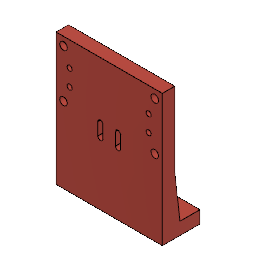
Y-endstop-holder-III-rev1 v6 (Autodesk Fusion 360 design; units mm, degrees)
Autodesk Fusion 360 part; units mm, degrees
note: some values were not read from the file. Set by a fixed rule: which sketch regions a step uses.
sketch "Sketch1" plane through (0, 0, 0) normal (0, 1, 0) x (1, 0, 0)
  line L0 (-21.15, 5) -> (21.15, 5)
  line L1 (21.15, 5) -> (21.15, -10)
  line L2 (21.15, -10) -> (-21.15, -10)
  line L3 (-21.15, -10) -> (-21.15, 5)
  line L4 (-15.5, 0) -> (15.5, 0) construction
  circle A0 centre (-15.5, 0) radius 1.5
  circle A1 centre (15.5, 0) radius 1.5
  circle A2 centre (0, 15.5) radius 14
  dimension "d1" = 42.3
  dimension "d2" = 15
  dimension "d3" = 31
  dimension "d4" = 5.65
  dimension "d5" = 3
  dimension "d6" = 3
  dimension "d9" = 28
  dimension "d13" = 15.5
  dimension "d14" = 5
  measures "d4" distance of origin
  measures "d5" diameter of A0
  measures "d6" diameter of A1
  measures "d9" diameter of A2
  measures "d14" distance of L0
extrude "Extrude1" add sketch "Sketch1" along normal blind 5 contours L0 L1 L2 L3 A2
sketch "Sketch2" plane through (0, 5, 0) normal (0, 1, 0) x (-1, 0, 0)
  line L0 (21.15, 5) -> (-21.15, 5)
  line L1 (-21.15, 5) -> (-21.15, 10)
  line L2 (-21.15, 10) -> (21.15, 10)
  line L3 (21.15, 10) -> (21.15, 5)
  circle A0 centre (-15.5, 0) radius 1.5
  circle A1 centre (15.5, 0) radius 1.5
  line L4 (-21.15, 10) -> (-21.15, -5)
  line L5 (-21.15, -5) -> (-9.2601, -5)
  arc A2 (9.2601, -5) -> (-9.2601, -5) centre (0, -15.5) ccw
  line L6 (9.2601, -5) -> (21.15, -5)
  line L7 (21.15, -5) -> (21.15, 10)
  line L8 (21.15, 10) -> (-21.15, 10)
  dimension "d22" = 5
  dimension "d23" = 42.3
extrude "Extrude2" add sketch "Sketch2" along normal blind 47.5 contours L0 L1 L2 L3 L4 L7 L8
sketch "Sketch3" plane through (0, 0, 5) normal (0, 0, -1) x (-1, 0, 0)
  line L0 (-15.7, 42.75) -> (-15.7, 36.25) construction
  circle A0 centre (-15.7, 42.75) radius 1
  circle A1 centre (-15.7, 36.25) radius 1
  line L1 (-21.15, 52.5) -> (21.15, 52.5)
  line L2 (0, 52.5) -> (0, 12.5) construction
  line L3 (-4.5, 30) -> (-4.5, 25)
  arc A2 (-4.5, 25) -> (-2.5, 25) centre (-3.5, 25) ccw
  line L4 (-2.5, 25) -> (-2.5, 30)
  arc A3 (-2.5, 30) -> (-4.5, 30) centre (-3.5, 30) ccw
  line L5 (-3.5, 30) -> (-3.5, 25) construction
  dimension "d26" = 6.5
  dimension "d27" = 2
  dimension "d28" = 2
  dimension "d30" = 5.45
  dimension "d32" = 2
  dimension "d33" = 5
  dimension "d34" = 3.5
  dimension "d35" = 25
  dimension "d51" = 42.75
  measures "d27" diameter of A0
  measures "d28" diameter of A1
  measures "d30" distance of origin
  measures "d32" distance of L3 L4
  measures "d34" distance of L2 L5
  measures "d35" distance of origin
  measures "d51" distance of origin
extrude "Extrude3" cut sketch "Sketch3" against normal through all
mirror "Mirror1" about plane through (0, 0, 0) normal (1, 0, 0) of "Extrude3"
sketch "Sketch4" plane through (0, 0, 5) normal (0, 0, -1) x (-1, 0, 0)
  circle A0 centre (15.7, 42.75) radius 1
  circle A1 centre (15.7, 36.25) radius 1
  circle A2 centre (-15.7, 42.75) radius 1
  circle A3 centre (-15.7, 36.25) radius 1
  circle A4 centre (15.7, 42.75) radius 2.5
  circle A5 centre (15.7, 36.25) radius 1
  circle A6 centre (15.7, 36.25) radius 2.5
  circle A7 centre (-15.7, 42.75) radius 2.5
  circle A8 centre (-15.7, 36.25) radius 2.5
  dimension "d37" = 5
  dimension "d38" = 5
  dimension "d39" = 5
  dimension "d40" = 5
  measures "d37" diameter of A7
  measures "d38" diameter of A8
  measures "d39" diameter of A4
  measures "d40" diameter of A6
chamfer "Chamfer1" distance 2 distance2 18 1 edges at (0, 5, 5) measured on face at (0, 5, 2.8333)
sketch "Sketch5" plane through (0, 0, 10) normal (0, 0, 1) x (1, 0, 0)
  line L0 (-18.125, 49.175) -> (-18.125, 30.175)
  circle A0 centre (-18.125, 49.175) radius 1.5
  circle A1 centre (-18.125, 30.175) radius 1.5
  line L1 (-21.15, 0) -> (-21.15, 52.5)
  circle A2 centre (-15.7, 42.75) radius 1
  dimension "d45" = 19
  dimension "d46" = 3
  dimension "d47" = 3
  dimension "d49" = 6.425
  dimension "d50" = 2.425
  measures "d46" diameter of A0
  measures "d47" diameter of A1
extrude "Extrude5" cut sketch "Sketch5" against normal through all contours A0 | A1
mirror "Mirror2" about plane through (0, 0, 0) normal (1, 0, 0) of "Extrude5"
